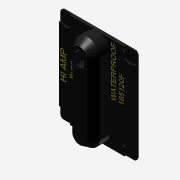
# Autodesk Inventor part: BUSS-COVER
Saved by Autodesk Inventor 2016 (Build 200138000, 138)
## iProperties
Shininess: 64.0
Length Units: 11272
Angle Units: 11279
Time Units: 11290
Mass Units: 11286
Length Display Precision: 3
Angle Display Precision: 2
Compacted: True
Part Number: BUSS-COVER
Document SubType Name: Modeling
Created: 2003-01-10
Designer: geyerm
Density: 1 g/cm^3
Material: Generic
Appearance: Glossy - Black
Mass: 7.12419 g
Surface Area: 49.8471 cm^2
Volume: 7.12419 cm^3
Density: 0.0
Volumn: 0.0
Area: 0.0
PropertySet Name: Model Information
Control State: 0
Master: False
Checked Out: False
Author: Autodesk
Autodesk Inventor part; units mm, degrees
ref_plane "YZ Plane" through (0, 0, 0) normal (1, 0, 0) x (0, 1, 0)
sketch "Sketch1" plane through (0, 0, 0) normal (0, 0, 1) x (1, 0, 0)
  arc A0 (-48.1199, -19.5796) -> (-46.5959, -21.1036) centre (-46.5959, -19.5796) ccw projected
  line L0 (-46.5959, -21.1036) -> (-10.7819, -21.1036) projected
  arc A1 (-10.7819, -21.1036) -> (-9.2579, -19.5796) centre (-10.7819, -19.5796) ccw projected
  line L1 (-9.2579, -19.5796) -> (-9.2579, 25.6324) projected
  arc A2 (-9.2579, 25.6324) -> (-10.7819, 27.1564) centre (-10.7819, 25.6324) ccw projected
  line L2 (-10.7819, 27.1564) -> (-46.5959, 27.1564) projected
  arc A3 (-46.5959, 27.1564) -> (-48.1199, 25.6324) centre (-46.5959, 25.6324) ccw projected
  line L3 (-48.1199, -19.5796) -> (-48.1199, 25.6324) projected
extrude "Extrusion1" add sketch "Sketch1" along normal blind 1.524
sketch "Sketch2" plane through (0, 0, 1.524) normal (0, 0, 1) x (1, 0, 0)
  line L0 (-10.7819, -21.1036) -> (-46.5959, -21.1036) projected
  line L1 (-46.5959, 27.1564) -> (-10.7819, 27.1564) projected
  line L2 (-35.0389, 20.8064) -> (-35.0389, -14.7536)
  arc A0 (-35.0389, -14.7536) -> (-22.3389, -14.7536) centre (-28.6889, -14.7536) ccw
  line L3 (-22.3389, -14.7536) -> (-22.3389, 20.8064)
  arc A1 (-22.3389, 20.8064) -> (-35.0389, 20.8064) centre (-28.6889, 20.8064) ccw
  line L4 (-28.6889, 27.1564) -> (-28.6889, -21.1036) construction
  dimension "d2" = 6.35
  constraints: 6 end point, 6 tangent, 4 point on circle, 2 centre point, 2 midpoint, 1 parallel, 1 point on line, 1 vertical
  measures "d2" radius of A1
extrude "Extrusion2" add sketch "Sketch2" along normal blind 8.89
chamfer "Chamfer2" distance 3.81 distance2 2.54 4 edges at (-35.0389, 3.0264, 10.414) (-28.6889, 27.1564, 10.414) (-22.3389, 3.0264, 10.414) (-28.6889, -21.1036, 10.414) measured on face at (-30.8056, 8.9531, 10.414) measured on face at (-35.0389, 8.9531, 4.4873)
sketch "Sketch3" plane through (0, 0, 10.414) normal (0, 0, 1) x (1, 0, 0)
  line L0 (-24.8789, 20.8064) -> (-24.8789, -14.7536) projected
  arc A0 (-24.8789, 20.8064) -> (-32.4989, 20.8064) centre (-28.6889, 20.8064) ccw projected
  line L1 (-30.8479, 20.8064) -> (-30.8479, 17.5044)
  arc A1 (-30.8479, 17.5044) -> (-26.5299, 17.5044) centre (-28.6889, 17.5044) ccw
  line L2 (-26.5299, 17.5044) -> (-26.5299, 20.8064)
  arc A2 (-26.5299, 20.8064) -> (-30.8479, 20.8064) centre (-28.6889, 20.8064) ccw
  dimension "d10" = 2.159
  dimension "d11" = 7.62
  constraints: 4 end point, 4 point on circle, 3 tangent, 2 centre point, 2 parallel, 1 coincident
  measures "d10" radius of A2
extrude "Extrusion3" cut sketch "Sketch3" against normal blind 8.89
ref_plane "Work Plane1" through (-48.1199, 3.0264, 0) normal (0, 1, 0) x (-1, 0, 0)
ref_plane "Work Plane2" through (-28.6889, 27.1564, 0) normal (1, 0, 0) x (0, 1, 0)
sketch "Sketch5" plane through (0, 0, 1.524) normal (0, 0, 1) x (1, 0, 0)
  line L0 (-35.0389, -14.7536) -> (-35.0389, 20.8064) projected
  line L1 (-46.5959, 27.1564) -> (-28.6889, 27.1564) projected
  arc A0 (-46.5959, 27.1564) -> (-48.1199, 25.6324) centre (-46.5959, 25.6324) ccw projected
  line L2 (-48.1199, -19.5796) -> (-48.1199, 25.6324) projected
  arc A1 (-47.0084, 21.5684) -> (-42.5319, 26.0449) centre (-44.9449, 23.9814) ccw
  line L3 (-41.7699, 23.9814) -> (-41.7699, 27.1564) construction
  line L4 (-44.9449, 20.8064) -> (-48.1199, 20.8064) construction
  line L5 (-47.0084, 21.5684) -> (-48.1199, 21.5684)
  line L6 (-42.5319, 26.0449) -> (-42.5319, 27.1564)
  dimension "d17" = 6.35
  dimension "d18" = 0.762
  dimension "d19" = 0.762
  constraints: 8 end point, 4 point on circle, 4 point on line, 4 tangent, 3 parallel, 1 centre point, 1 perpendicular
  measures "d17" diameter of A1
  measures "d18" distance between parallel lines of L6 L3
  measures "d19" distance between parallel lines of L5 L4
extrude "Extrusion5" cut sketch "Sketch5" against normal blind 0.762
mirror "Mirror3" about plane through (-48.1199, 3.0264, 0) normal (0, 1, 0) of "Extrusion5"
mirror "Mirror4" about plane through (-28.6889, 27.1564, 0) normal (1, 0, 0) of "Extrusion5", "Mirror3"
sketch "Sketch6" plane through (0, 0, 1.524) normal (0, 0, 1) x (1, 0, 0)
  line L0 (-48.1199, -15.5156) -> (-48.1199, 21.5684) projected
  line L1 (-47.3926, -5.3988) -> (-47.3926, 12.5954) construction
  line L2 (-47.3926, 12.5954) -> (-36.8812, 12.5954) construction
  line L3 (-36.8812, 12.5954) -> (-36.8812, -5.3988) construction
  line L4 (-36.8812, -5.3988) -> (-47.3926, -5.3988) construction
  line L5 (-44.3446, -3.3933) -> (-47.3926, -3.3933)
  line L6 (-47.3926, -3.3933) -> (-47.3926, -2.9891)
  line L7 (-47.3926, -2.9891) -> (-46.1404, -2.9891)
  line L8 (-46.1404, -2.9891) -> (-46.1404, -1.4093)
  line L9 (-46.1404, -1.4093) -> (-47.3926, -1.4093)
  line L10 (-47.3926, -1.4093) -> (-47.3926, -1.0051)
  line L11 (-47.3926, -1.0051) -> (-44.3446, -1.0051)
  line L12 (-44.3446, -1.0051) -> (-44.3446, -1.4093)
  line L13 (-44.3446, -1.4093) -> (-45.7803, -1.4093)
  line L14 (-45.7803, -1.4093) -> (-45.7803, -2.9891)
  line L15 (-45.7803, -2.9891) -> (-44.3446, -2.9891)
  line L16 (-44.3446, -2.9891) -> (-44.3446, -3.3933)
  line L17 (-44.3446, -0.264) -> (-47.3926, -0.264)
  line L18 (-47.3926, -0.264) -> (-47.3926, 0.1403)
  line L19 (-47.3926, 0.1403) -> (-44.3446, 0.1403)
  line L20 (-44.3446, 0.1403) -> (-44.3446, -0.264)
  line L21 (-44.3446, 1.6991) -> (-47.3926, 2.87)
  line L22 (-47.3926, 2.87) -> (-47.3926, 3.3067)
  line L23 (-47.3926, 3.3067) -> (-44.3446, 4.552)
  line L24 (-44.3446, 4.552) -> (-44.3446, 4.092)
  line L25 (-44.3446, 4.092) -> (-45.2669, 3.7388)
  line L26 (-45.2669, 3.7388) -> (-45.2669, 2.4611)
  line L27 (-45.2669, 2.4611) -> (-44.3446, 2.1266)
  line L28 (-44.3446, 2.1266) -> (-44.3446, 1.6991)
  line L29 (-45.5945, 2.5773) -> (-45.5945, 3.6134)
  line L30 (-45.5945, 3.6134) -> (-46.4401, 3.2928)
  spline S0 degree 2 poles (-46.4401, 3.2928) (-46.8257, 3.1488) (-47.072, 3.0791) knots 0 0 0 1 1 1
  spline S1 degree 2 poles (-47.072, 3.0791) (-46.7793, 3.0187) (-46.4889, 2.9141) knots 0 0 0 1 1 1
  line L31 (-46.4889, 2.9141) -> (-45.5945, 2.5773)
  line L32 (-44.3446, 4.8609) -> (-47.3926, 4.8609)
  line L33 (-47.3926, 4.8609) -> (-47.3926, 5.4673)
  line L34 (-47.3926, 5.4673) -> (-45.2344, 6.1898)
  spline S2 degree 2 poles (-45.2344, 6.1898) (-44.9324, 6.2897) (-44.7837, 6.3361) knots 0 0 0 1 1 1
  spline S3 degree 2 poles (-44.7837, 6.3361) (-44.9486, 6.3873) (-45.2715, 6.4988) knots 0 0 0 1 1 1
  line L35 (-45.2715, 6.4988) -> (-47.3926, 7.2306)
  line L36 (-47.3926, 7.2306) -> (-47.3926, 7.7719)
  line L37 (-47.3926, 7.7719) -> (-44.3446, 7.7719)
  line L38 (-44.3446, 7.7719) -> (-44.3446, 7.3839)
  line L39 (-44.3446, 7.3839) -> (-46.8954, 7.3839)
  line L40 (-46.8954, 7.3839) -> (-44.3446, 6.4941)
  line L41 (-44.3446, 6.4941) -> (-44.3446, 6.1317)
  line L42 (-44.3446, 6.1317) -> (-46.9396, 5.2489)
  line L43 (-46.9396, 5.2489) -> (-44.3446, 5.2489)
  line L44 (-44.3446, 5.2489) -> (-44.3446, 4.8609)
  line L45 (-44.3446, 8.42) -> (-47.3926, 8.42)
  line L46 (-47.3926, 8.42) -> (-47.3926, 9.57)
  spline S4 degree 2 poles (-47.3926, 9.57) (-47.3926, 9.8743) (-47.3624, 10.0346) knots 0 0 0 1 1 1
  spline S5 degree 4 poles (-47.3624, 10.0346) (-47.3252, 10.26) (-47.1161, 10.562) (-46.7375, 10.7478) (-46.5098, 10.7478) knots 0 0 0 0 0 1 1 1 1 1
  spline S6 degree 3 poles (-46.5098, 10.7478) (-46.1218, 10.7478) (-45.5829, 10.253) (-45.5829, 9.6072) knots 0 0 0 0 1 1 1 1
  line L47 (-45.5829, 9.6072) -> (-45.5829, 8.8243)
  line L48 (-45.5829, 8.8243) -> (-44.3446, 8.8243)
  line L49 (-44.3446, 8.8243) -> (-44.3446, 8.42)
  line L50 (-45.9429, 8.8243) -> (-45.9429, 9.6118)
  spline S7 degree 3 poles (-45.9429, 9.6118) (-45.9429, 10.0044) (-46.2333, 10.332) (-46.4982, 10.332) knots 0 0 0 0 1 1 1 1
  spline S8 degree 3 poles (-46.4982, 10.332) (-46.6887, 10.332) (-46.9628, 10.1392) (-47.0046, 9.9812) knots 0 0 0 0 1 1 1 1
  spline S9 degree 2 poles (-47.0046, 9.9812) (-47.0325, 9.879) (-47.0325, 9.6048) knots 0 0 0 1 1 1
  line L51 (-47.0325, 9.6048) -> (-47.0325, 8.8243)
  line L52 (-47.0325, 8.8243) -> (-45.9429, 8.8243)
  line L53 (-40.1526, -0.0878) -> (-42.6926, -0.0878)
  line L54 (-42.6926, -0.0878) -> (-42.6926, 0.8647)
  spline S10 degree 4 poles (-42.6926, 0.8647) (-42.6926, 1.1551) (-42.5378, 1.5074) (-42.2183, 1.7068) (-42.0421, 1.7068) knots 0 0 0 0 0 1 1 1 1 1
  spline S11 degree 3 poles (-42.0421, 1.7068) (-41.8795, 1.7068) (-41.593, 1.5307) (-41.5039, 1.3506) knots 0 0 0 0 1 1 1 1
  spline S12 degree 3 poles (-41.5039, 1.3506) (-41.4362, 1.5829) (-41.1109, 1.8307) (-40.8883, 1.8307) knots 0 0 0 0 1 1 1 1
  spline S13 degree 5 poles (-40.8883, 1.8307) (-40.7102, 1.8307) (-40.4043, 1.6797) (-40.2378, 1.459) (-40.1526, 1.1241) (-40.1526, 0.8802) knots 0 0 0 0 0 0 1 1 1 1 1 1
  line L55 (-40.1526, 0.8802) -> (-40.1526, -0.0878)
  line L56 (-40.4527, 0.2491) -> (-40.4527, 0.8821)
  spline S14 degree 2 poles (-40.4527, 0.8821) (-40.4527, 1.0447) (-40.4643, 1.1106) knots 0 0 0 1 1 1
  spline S15 degree 4 poles (-40.4643, 1.1106) (-40.4856, 1.2267) (-40.5824, 1.3835) (-40.7683, 1.4842) (-40.8902, 1.4842) knots 0 0 0 0 0 1 1 1 1 1
  spline S16 degree 4 poles (-40.8902, 1.4842) (-41.0316, 1.4842) (-41.2407, 1.3351) (-41.3258, 1.0776) (-41.3258, 0.8357) knots 0 0 0 0 0 1 1 1 1 1
  line L57 (-41.3258, 0.8357) -> (-41.3258, 0.2491)
  line L58 (-41.3258, 0.2491) -> (-40.4527, 0.2491)
  line L59 (-41.6259, 0.2491) -> (-41.6259, 0.7969)
  spline S17 degree 2 poles (-41.6259, 0.7969) (-41.6259, 1.0215) (-41.655, 1.1183) knots 0 0 0 1 1 1
  spline S18 degree 3 poles (-41.655, 1.1183) (-41.6937, 1.2461) (-41.8698, 1.3758) (-42.0034, 1.3758) knots 0 0 0 0 1 1 1 1
  spline S19 degree 4 poles (-42.0034, 1.3758) (-42.1293, 1.3758) (-42.3209, 1.2538) (-42.3926, 1.0293) (-42.3926, 0.7563) knots 0 0 0 0 0 1 1 1 1 1
  line L60 (-42.3926, 0.7563) -> (-42.3926, 0.2491)
  line L61 (-42.3926, 0.2491) -> (-41.6259, 0.2491)
  line L62 (-40.1526, 3.4589) -> (-40.4237, 3.4589)
  spline S20 degree 2 poles (-40.4237, 3.4589) (-40.112, 3.244) (-40.112, 2.8762) knots 0 0 0 1 1 1
  spline S21 degree 4 poles (-40.112, 2.8762) (-40.112, 2.7135) (-40.2359, 2.4309) (-40.4256, 2.2934) (-40.5631, 2.2663) knots 0 0 0 0 0 1 1 1 1 1
  spline S22 degree 2 poles (-40.5631, 2.2663) (-40.6541, 2.247) (-40.8535, 2.247) knots 0 0 0 1 1 1
  line L63 (-40.8535, 2.247) -> (-41.9937, 2.247)
  line L64 (-41.9937, 2.247) -> (-41.9937, 2.5587)
  line L65 (-41.9937, 2.5587) -> (-40.9735, 2.5587)
  spline S23 degree 2 poles (-40.9735, 2.5587) (-40.7296, 2.5587) (-40.6444, 2.578) knots 0 0 0 1 1 1
  spline S24 degree 3 poles (-40.6444, 2.578) (-40.5205, 2.6071) (-40.3811, 2.7968) (-40.3811, 2.9381) knots 0 0 0 0 1 1 1 1
  spline S25 degree 4 poles (-40.3811, 2.9381) (-40.3811, 3.0775) (-40.5243, 3.3234) (-40.7721, 3.426) (-41.0083, 3.426) knots 0 0 0 0 0 1 1 1 1 1
  line L66 (-41.0083, 3.426) -> (-41.9937, 3.426)
  line L67 (-41.9937, 3.426) -> (-41.9937, 3.7377)
  line L68 (-41.9937, 3.7377) -> (-40.1526, 3.7377)
  line L69 (-40.1526, 3.7377) -> (-40.1526, 3.4589)
  line L70 (-40.7025, 4.1016) -> (-40.7509, 4.4095)
  spline S26 degree 3 poles (-40.7509, 4.4095) (-40.565, 4.4346) (-40.3675, 4.6728) (-40.3675, 4.8876) knots 0 0 0 0 1 1 1 1
  spline S27 degree 3 poles (-40.3675, 4.8876) (-40.3675, 5.1025) (-40.5437, 5.3116) (-40.6618, 5.3116) knots 0 0 0 0 1 1 1 1
  spline S28 degree 2 poles (-40.6618, 5.3116) (-40.7663, 5.3116) (-40.8283, 5.2187) knots 0 0 0 1 1 1
  spline S29 degree 2 poles (-40.8283, 5.2187) (-40.8689, 5.1548) (-40.9328, 4.8993) knots 0 0 0 1 1 1
  spline S30 degree 4 poles (-40.9328, 4.8993) (-41.02, 4.5566) (-41.1458, 4.2914) (-41.3704, 4.1539) (-41.5039, 4.1539) knots 0 0 0 0 0 1 1 1 1 1
  spline S31 degree 3 poles (-41.5039, 4.1539) (-41.6278, 4.1539) (-41.8369, 4.2662) (-41.9066, 4.363) knots 0 0 0 0 1 1 1 1
  spline S32 degree 3 poles (-41.9066, 4.363) (-41.9608, 4.4366) (-42.0344, 4.6882) (-42.0344, 4.8334) knots 0 0 0 0 1 1 1 1
  spline S33 degree 4 poles (-42.0344, 4.8334) (-42.0344, 5.0503) (-41.9086, 5.3775) (-41.6956, 5.5343) (-41.5175, 5.5633) knots 0 0 0 0 0 1 1 1 1 1
  line L71 (-41.5175, 5.5633) -> (-41.4768, 5.2574)
  spline S34 degree 3 poles (-41.4768, 5.2574) (-41.6201, 5.2361) (-41.7789, 5.0367) (-41.7789, 4.8547) knots 0 0 0 0 1 1 1 1
  spline S35 degree 3 poles (-41.7789, 4.8547) (-41.7789, 4.6398) (-41.6356, 4.4559) (-41.5407, 4.4559) knots 0 0 0 0 1 1 1 1
  spline S36 degree 2 poles (-41.5407, 4.4559) (-41.4807, 4.4559) (-41.4323, 4.4946) knots 0 0 0 1 1 1
  spline S37 degree 2 poles (-41.4323, 4.4946) (-41.382, 4.5314) (-41.3491, 4.6147) knots 0 0 0 1 1 1
  spline S38 degree 2 poles (-41.3491, 4.6147) (-41.3316, 4.6611) (-41.2678, 4.8896) knots 0 0 0 1 1 1
  spline S39 degree 4 poles (-41.2678, 4.8896) (-41.1806, 5.2206) (-41.0684, 5.4839) (-40.8535, 5.633) (-40.6928, 5.633) knots 0 0 0 0 0 1 1 1 1 1
  spline S40 degree 4 poles (-40.6928, 5.633) (-40.5379, 5.633) (-40.263, 5.451) (-40.112, 5.1064) (-40.112, 4.8896) knots 0 0 0 0 0 1 1 1 1 1
  spline S41 degree 3 poles (-40.112, 4.8896) (-40.112, 4.5314) (-40.4101, 4.1539) (-40.7025, 4.1016) knots 0 0 0 0 1 1 1 1
  line L72 (-40.7025, 5.8769) -> (-40.7509, 6.1848)
  spline S42 degree 3 poles (-40.7509, 6.1848) (-40.565, 6.2099) (-40.3675, 6.448) (-40.3675, 6.6629) knots 0 0 0 0 1 1 1 1
  spline S43 degree 3 poles (-40.3675, 6.6629) (-40.3675, 6.8778) (-40.5437, 7.0869) (-40.6618, 7.0869) knots 0 0 0 0 1 1 1 1
  spline S44 degree 2 poles (-40.6618, 7.0869) (-40.7663, 7.0869) (-40.8283, 6.994) knots 0 0 0 1 1 1
  spline S45 degree 2 poles (-40.8283, 6.994) (-40.8689, 6.9301) (-40.9328, 6.6746) knots 0 0 0 1 1 1
  spline S46 degree 4 poles (-40.9328, 6.6746) (-41.02, 6.3319) (-41.1458, 6.0667) (-41.3704, 5.9292) (-41.5039, 5.9292) knots 0 0 0 0 0 1 1 1 1 1
  spline S47 degree 3 poles (-41.5039, 5.9292) (-41.6278, 5.9292) (-41.8369, 6.0415) (-41.9066, 6.1383) knots 0 0 0 0 1 1 1 1
  spline S48 degree 3 poles (-41.9066, 6.1383) (-41.9608, 6.2119) (-42.0344, 6.4635) (-42.0344, 6.6087) knots 0 0 0 0 1 1 1 1
  spline S49 degree 4 poles (-42.0344, 6.6087) (-42.0344, 6.8256) (-41.9086, 7.1527) (-41.6956, 7.3096) (-41.5175, 7.3386) knots 0 0 0 0 0 1 1 1 1 1
  line L73 (-41.5175, 7.3386) -> (-41.4768, 7.0327)
  spline S50 degree 3 poles (-41.4768, 7.0327) (-41.6201, 7.0114) (-41.7789, 6.812) (-41.7789, 6.63) knots 0 0 0 0 1 1 1 1
  spline S51 degree 3 poles (-41.7789, 6.63) (-41.7789, 6.4151) (-41.6356, 6.2312) (-41.5407, 6.2312) knots 0 0 0 0 1 1 1 1
  spline S52 degree 2 poles (-41.5407, 6.2312) (-41.4807, 6.2312) (-41.4323, 6.2699) knots 0 0 0 1 1 1
  spline S53 degree 2 poles (-41.4323, 6.2699) (-41.382, 6.3067) (-41.3491, 6.39) knots 0 0 0 1 1 1
  spline S54 degree 2 poles (-41.3491, 6.39) (-41.3316, 6.4364) (-41.2678, 6.6649) knots 0 0 0 1 1 1
  spline S55 degree 4 poles (-41.2678, 6.6649) (-41.1806, 6.9959) (-41.0684, 7.2592) (-40.8535, 7.4083) (-40.6928, 7.4083) knots 0 0 0 0 0 1 1 1 1 1
  spline S56 degree 4 poles (-40.6928, 7.4083) (-40.5379, 7.4083) (-40.263, 7.2263) (-40.112, 6.8817) (-40.112, 6.6649) knots 0 0 0 0 0 1 1 1 1 1
  spline S57 degree 3 poles (-40.112, 6.6649) (-40.112, 6.3067) (-40.4101, 5.9292) (-40.7025, 5.8769) knots 0 0 0 0 1 1 1 1
  line L74 (-36.1554, 0.7708) -> (-36.1554, 0.4591)
  line L75 (-36.1554, 0.4591) -> (-38.1417, 0.4591)
  spline S58 degree 3 poles (-38.1417, 0.4591) (-38.0353, 0.3468) (-37.8204, -0.0191) (-37.7662, -0.1643) knots 0 0 0 0 1 1 1 1
  line L76 (-37.7662, -0.1643) -> (-38.0682, -0.1643)
  spline S59 degree 3 poles (-38.0682, -0.1643) (-38.1901, 0.0971) (-38.5406, 0.4881) (-38.7051, 0.5695) knots 0 0 0 0 1 1 1 1
  line L77 (-38.7051, 0.5695) -> (-38.7051, 0.7708)
  line L78 (-38.7051, 0.7708) -> (-36.1554, 0.7708)
  line L79 (-36.4555, 3.2082) -> (-36.1554, 3.2082)
  line L80 (-36.1554, 3.2082) -> (-36.1554, 1.5297)
  spline S60 degree 2 poles (-36.1554, 1.5297) (-36.2677, 1.5258) (-36.3723, 1.5665) knots 0 0 0 1 1 1
  spline S61 degree 3 poles (-36.3723, 1.5665) (-36.5446, 1.6304) (-36.8756, 1.913) (-37.0944, 2.1802) knots 0 0 0 0 1 1 1 1
  spline S62 degree 3 poles (-37.0944, 2.1802) (-37.4351, 2.5926) (-37.83, 2.8829) (-38.0082, 2.8829) knots 0 0 0 0 1 1 1 1
  spline S63 degree 3 poles (-38.0082, 2.8829) (-38.194, 2.8829) (-38.4476, 2.6177) (-38.4476, 2.4048) knots 0 0 0 0 1 1 1 1
  spline S64 degree 3 poles (-38.4476, 2.4048) (-38.4476, 2.1802) (-38.1766, 1.9111) (-37.9385, 1.9092) knots 0 0 0 0 1 1 1 1
  line L81 (-37.9385, 1.9092) -> (-37.9714, 1.5878)
  spline S65 degree 3 poles (-37.9714, 1.5878) (-38.3295, 1.6207) (-38.7051, 2.0505) (-38.7051, 2.4125) knots 0 0 0 0 1 1 1 1
  spline S66 degree 3 poles (-38.7051, 2.4125) (-38.7051, 2.7784) (-38.3005, 3.2043) (-38.0004, 3.2043) knots 0 0 0 0 1 1 1 1
  spline S67 degree 4 poles (-38.0004, 3.2043) (-37.8475, 3.2043) (-37.5532, 3.0804) (-37.228, 2.79) (-36.9434, 2.4551) knots 0 0 0 0 0 1 1 1 1 1
  spline S68 degree 3 poles (-36.9434, 2.4551) (-36.7091, 2.1744) (-36.5407, 2.0156) (-36.4555, 1.9634) knots 0 0 0 0 1 1 1 1
  line L82 (-36.4555, 1.9634) -> (-36.4555, 3.2082)
  spline S69 degree 4 poles (-37.408, 3.5431) (-37.8591, 3.5431) (-38.4089, 3.729) (-38.7051, 4.0929) (-38.7051, 4.3717) knots 0 0 0 0 0 1 1 1 1 1
  spline S70 degree 5 poles (-38.7051, 4.3717) (-38.7051, 4.575) (-38.5406, 4.8847) (-38.2308, 5.0842) (-37.7855, 5.1984) (-37.408, 5.1984) knots 0 0 0 0 0 0 1 1 1 1 1 1
  spline S71 degree 4 poles (-37.408, 5.1984) (-36.9608, 5.1984) (-36.411, 5.0145) (-36.1128, 4.6486) (-36.1128, 4.3717) knots 0 0 0 0 0 1 1 1 1 1
  spline S72 degree 2 poles (-36.1128, 4.3717) (-36.1128, 4.0039) (-36.3742, 3.7948) knots 0 0 0 1 1 1
  spline S73 degree 2 poles (-36.3742, 3.7948) (-36.6936, 3.5431) (-37.408, 3.5431) knots 0 0 0 1 1 1
  spline S74 degree 3 poles (-37.408, 3.8645) (-36.7808, 3.8645) (-36.3684, 4.1568) (-36.3684, 4.3717) knots 0 0 0 0 1 1 1 1
  spline S75 degree 3 poles (-36.3684, 4.3717) (-36.3684, 4.5847) (-36.7827, 4.877) (-37.408, 4.877) knots 0 0 0 0 1 1 1 1
  spline S76 degree 3 poles (-37.408, 4.877) (-38.0353, 4.877) (-38.4476, 4.5847) (-38.4476, 4.3678) knots 0 0 0 0 1 1 1 1
  spline S77 degree 2 poles (-38.4476, 4.3678) (-38.4476, 4.1529) (-38.2656, 4.0252) knots 0 0 0 1 1 1
  spline S78 degree 2 poles (-38.2656, 4.0252) (-38.0333, 3.8645) (-37.408, 3.8645) knots 0 0 0 1 1 1
  line L83 (-36.1554, 5.3649) -> (-38.6954, 6.3406)
  line L84 (-38.6954, 6.3406) -> (-38.6954, 6.7046)
  line L85 (-38.6954, 6.7046) -> (-36.1554, 7.7422)
  line L86 (-36.1554, 7.7422) -> (-36.1554, 7.3589)
  line L87 (-36.1554, 7.3589) -> (-36.924, 7.0647)
  line L88 (-36.924, 7.0647) -> (-36.924, 5.9999)
  line L89 (-36.924, 5.9999) -> (-36.1554, 5.7211)
  line L90 (-36.1554, 5.7211) -> (-36.1554, 5.3649)
  line L91 (-37.197, 6.0967) -> (-37.197, 6.9601)
  line L92 (-37.197, 6.9601) -> (-37.9017, 6.6929)
  spline S79 degree 2 poles (-37.9017, 6.6929) (-38.2231, 6.5729) (-38.4283, 6.5148) knots 0 0 0 1 1 1
  spline S80 degree 2 poles (-38.4283, 6.5148) (-38.1843, 6.4645) (-37.9423, 6.3774) knots 0 0 0 1 1 1
  line L93 (-37.9423, 6.3774) -> (-37.197, 6.0967)
  constraints: 1 parallel, 2 other
emboss "Emboss1" sketch "Sketch6" operation add depth 0.0508 direction (0, 0, -1)
sketch "Sketch7" plane through (0, 0, 1.524) normal (0, 0, 1) x (1, 0, 0)
  line L0 (-9.2579, 21.5684) -> (-9.2579, -15.5156) projected
  line L1 (-21.7032, 0.6221) -> (-21.7032, 0.6221) construction
  line L2 (-21.7032, 0.6221) -> (-21.7032, 0.6221) construction
  line L3 (-21.7032, 0.6221) -> (-21.7032, 0.6221) construction
  line L4 (-21.7032, 0.6221) -> (-21.7032, 0.6221) construction
  line L5 (-19.1186, 1.3384) -> (-21.6586, 0.6647)
  line L6 (-21.6586, 0.6647) -> (-21.6586, 1.0093)
  line L7 (-21.6586, 1.0093) -> (-19.9937, 1.3965)
  spline S0 degree 2 poles (-19.9937, 1.3965) (-19.7323, 1.4584) (-19.4729, 1.5049) knots 0 0 0 1 1 1
  spline S1 degree 2 poles (-19.4729, 1.5049) (-19.8814, 1.6017) (-19.9434, 1.6191) knots 0 0 0 1 1 1
  line L8 (-19.9434, 1.6191) -> (-21.6586, 2.1012)
  line L9 (-21.6586, 2.1012) -> (-21.6586, 2.5077)
  line L10 (-21.6586, 2.5077) -> (-20.3732, 2.8717)
  spline S2 degree 2 poles (-20.3732, 2.8717) (-19.895, 3.0053) (-19.4729, 3.0692) knots 0 0 0 1 1 1
  spline S3 degree 2 poles (-19.4729, 3.0692) (-19.7149, 3.1176) (-20.0266, 3.195) knots 0 0 0 1 1 1
  line L11 (-20.0266, 3.195) -> (-21.6586, 3.5919)
  line L12 (-21.6586, 3.5919) -> (-21.6586, 3.9307)
  line L13 (-21.6586, 3.9307) -> (-19.1186, 3.2376)
  line L14 (-19.1186, 3.2376) -> (-19.1186, 2.9085)
  line L15 (-19.1186, 2.9085) -> (-21.0546, 2.378)
  spline S4 degree 2 poles (-21.0546, 2.378) (-21.2966, 2.3083) (-21.3528, 2.2967) knots 0 0 0 1 1 1
  spline S5 degree 2 poles (-21.3528, 2.2967) (-21.1785, 2.2541) (-21.0546, 2.2212) knots 0 0 0 1 1 1
  line L16 (-21.0546, 2.2212) -> (-19.1186, 1.6849)
  line L17 (-19.1186, 1.6849) -> (-19.1186, 1.3384)
  line L18 (-19.1186, 3.9674) -> (-21.6586, 4.9432)
  line L19 (-21.6586, 4.9432) -> (-21.6586, 5.3071)
  line L20 (-21.6586, 5.3071) -> (-19.1186, 6.3448)
  line L21 (-19.1186, 6.3448) -> (-19.1186, 5.9615)
  line L22 (-19.1186, 5.9615) -> (-19.8872, 5.6672)
  line L23 (-19.8872, 5.6672) -> (-19.8872, 4.6024)
  line L24 (-19.8872, 4.6024) -> (-19.1186, 4.3237)
  line L25 (-19.1186, 4.3237) -> (-19.1186, 3.9674)
  line L26 (-20.1602, 4.6992) -> (-20.1602, 5.5627)
  line L27 (-20.1602, 5.5627) -> (-20.8649, 5.2955)
  spline S6 degree 2 poles (-20.8649, 5.2955) (-21.1863, 5.1755) (-21.3915, 5.1174) knots 0 0 0 1 1 1
  spline S7 degree 2 poles (-21.3915, 5.1174) (-21.1475, 5.0671) (-20.9055, 4.98) knots 0 0 0 1 1 1
  line L28 (-20.9055, 4.98) -> (-20.1602, 4.6992)
  line L29 (-19.1186, 7.2586) -> (-21.3586, 7.2586)
  line L30 (-21.3586, 7.2586) -> (-21.3586, 6.4223)
  line L31 (-21.3586, 6.4223) -> (-21.6586, 6.4223)
  line L32 (-21.6586, 6.4223) -> (-21.6586, 8.4357)
  line L33 (-21.6586, 8.4357) -> (-21.3586, 8.4357)
  line L34 (-21.3586, 8.4357) -> (-21.3586, 7.5955)
  line L35 (-21.3586, 7.5955) -> (-19.1186, 7.5955)
  line L36 (-19.1186, 7.5955) -> (-19.1186, 7.2586)
  line L37 (-19.1186, 8.788) -> (-21.6586, 8.788)
  line L38 (-21.6586, 8.788) -> (-21.6586, 10.6272)
  line L39 (-21.6586, 10.6272) -> (-21.3586, 10.6272)
  line L40 (-21.3586, 10.6272) -> (-21.3586, 9.1249)
  line L41 (-21.3586, 9.1249) -> (-20.5822, 9.1249)
  line L42 (-20.5822, 9.1249) -> (-20.5822, 10.5323)
  line L43 (-20.5822, 10.5323) -> (-20.2822, 10.5323)
  line L44 (-20.2822, 10.5323) -> (-20.2822, 9.1249)
  line L45 (-20.2822, 9.1249) -> (-19.4187, 9.1249)
  line L46 (-19.4187, 9.1249) -> (-19.4187, 10.6853)
  line L47 (-19.4187, 10.6853) -> (-19.1186, 10.6853)
  line L48 (-19.1186, 10.6853) -> (-19.1186, 8.788)
  line L49 (-19.1186, 11.1538) -> (-21.6586, 11.1538)
  line L50 (-21.6586, 11.1538) -> (-21.6586, 12.2805)
  spline S8 degree 4 poles (-21.6586, 12.2805) (-21.6586, 12.6193) (-21.5212, 12.9736) (-21.1746, 13.1846) (-20.9656, 13.1846) knots 0 0 0 0 0 1 1 1 1 1
  spline S9 degree 3 poles (-20.9656, 13.1846) (-20.6945, 13.1846) (-20.3248, 12.8342) (-20.2744, 12.4703) knots 0 0 0 0 1 1 1 1
  spline S10 degree 2 poles (-20.2744, 12.4703) (-20.2105, 12.6019) (-20.1486, 12.6716) knots 0 0 0 1 1 1
  spline S11 degree 2 poles (-20.1486, 12.6716) (-20.0131, 12.8187) (-19.8098, 12.9504) knots 0 0 0 1 1 1
  line L51 (-19.8098, 12.9504) -> (-19.1186, 13.3898)
  line L52 (-19.1186, 13.3898) -> (-19.1186, 12.9697)
  line L53 (-19.1186, 12.9697) -> (-19.6472, 12.6329)
  spline S12 degree 4 poles (-19.6472, 12.6329) (-19.8756, 12.4857) (-20.1176, 12.296) (-20.2163, 12.145) (-20.2357, 12.0676) knots 0 0 0 0 0 1 1 1 1 1
  spline S13 degree 2 poles (-20.2357, 12.0676) (-20.2473, 12.0095) (-20.2473, 11.8798) knots 0 0 0 1 1 1
  line L54 (-20.2473, 11.8798) -> (-20.2473, 11.4906)
  line L55 (-20.2473, 11.4906) -> (-19.1186, 11.4906)
  line L56 (-19.1186, 11.4906) -> (-19.1186, 11.1538)
  line L57 (-20.5377, 11.4906) -> (-20.5377, 12.2128)
  spline S14 degree 4 poles (-20.5377, 12.2128) (-20.5377, 12.4431) (-20.6326, 12.7026) (-20.8436, 12.8381) (-20.9656, 12.8381) knots 0 0 0 0 0 1 1 1 1 1
  spline S15 degree 3 poles (-20.9656, 12.8381) (-21.1456, 12.8381) (-21.3779, 12.5767) (-21.3779, 12.2941) knots 0 0 0 0 1 1 1 1
  line L58 (-21.3779, 12.2941) -> (-21.3779, 11.4906)
  line L59 (-21.3779, 11.4906) -> (-20.5377, 11.4906)
  line L60 (-19.1186, 13.7112) -> (-21.6586, 13.7112)
  line L61 (-21.6586, 13.7112) -> (-21.6586, 14.6695)
  spline S16 degree 2 poles (-21.6586, 14.6695) (-21.6586, 14.9231) (-21.6335, 15.0567) knots 0 0 0 1 1 1
  spline S17 degree 4 poles (-21.6335, 15.0567) (-21.6025, 15.2445) (-21.4283, 15.4962) (-21.1127, 15.6511) (-20.923, 15.6511) knots 0 0 0 0 0 1 1 1 1 1
  spline S18 degree 3 poles (-20.923, 15.6511) (-20.5997, 15.6511) (-20.1505, 15.2387) (-20.1505, 14.7005) knots 0 0 0 0 1 1 1 1
  line L62 (-20.1505, 14.7005) -> (-20.1505, 14.0481)
  line L63 (-20.1505, 14.0481) -> (-19.1186, 14.0481)
  line L64 (-19.1186, 14.0481) -> (-19.1186, 13.7112)
  line L65 (-20.4506, 14.0481) -> (-20.4506, 14.7044)
  spline S19 degree 3 poles (-20.4506, 14.7044) (-20.4506, 15.0315) (-20.6926, 15.3045) (-20.9133, 15.3045) knots 0 0 0 0 1 1 1 1
  spline S20 degree 3 poles (-20.9133, 15.3045) (-21.072, 15.3045) (-21.3005, 15.1438) (-21.3353, 15.0122) knots 0 0 0 0 1 1 1 1
  spline S21 degree 2 poles (-21.3353, 15.0122) (-21.3586, 14.927) (-21.3586, 14.6986) knots 0 0 0 1 1 1
  line L66 (-21.3586, 14.6986) -> (-21.3586, 14.0481)
  line L67 (-21.3586, 14.0481) -> (-20.4506, 14.0481)
  line L68 (-19.1186, 16.0847) -> (-21.6586, 16.0847)
  line L69 (-21.6586, 16.0847) -> (-21.6586, 17.2115)
  spline S22 degree 4 poles (-21.6586, 17.2115) (-21.6586, 17.5503) (-21.5212, 17.9045) (-21.1746, 18.1156) (-20.9656, 18.1156) knots 0 0 0 0 0 1 1 1 1 1
  spline S23 degree 3 poles (-20.9656, 18.1156) (-20.6945, 18.1156) (-20.3248, 17.7651) (-20.2744, 17.4012) knots 0 0 0 0 1 1 1 1
  spline S24 degree 2 poles (-20.2744, 17.4012) (-20.2105, 17.5328) (-20.1486, 17.6025) knots 0 0 0 1 1 1
  spline S25 degree 2 poles (-20.1486, 17.6025) (-20.0131, 17.7497) (-19.8098, 17.8813) knots 0 0 0 1 1 1
  line L70 (-19.8098, 17.8813) -> (-19.1186, 18.3208)
  line L71 (-19.1186, 18.3208) -> (-19.1186, 17.9007)
  line L72 (-19.1186, 17.9007) -> (-19.6472, 17.5638)
  spline S26 degree 4 poles (-19.6472, 17.5638) (-19.8756, 17.4167) (-20.1176, 17.2269) (-20.2163, 17.0759) (-20.2357, 16.9985) knots 0 0 0 0 0 1 1 1 1 1
  spline S27 degree 2 poles (-20.2357, 16.9985) (-20.2473, 16.9404) (-20.2473, 16.8107) knots 0 0 0 1 1 1
  line L73 (-20.2473, 16.8107) -> (-20.2473, 16.4216)
  line L74 (-20.2473, 16.4216) -> (-19.1186, 16.4216)
  line L75 (-19.1186, 16.4216) -> (-19.1186, 16.0847)
  line L76 (-20.5377, 16.4216) -> (-20.5377, 17.1437)
  spline S28 degree 4 poles (-20.5377, 17.1437) (-20.5377, 17.3741) (-20.6326, 17.6335) (-20.8436, 17.769) (-20.9656, 17.769) knots 0 0 0 0 0 1 1 1 1 1
  spline S29 degree 3 poles (-20.9656, 17.769) (-21.1456, 17.769) (-21.3779, 17.5077) (-21.3779, 17.225) knots 0 0 0 0 1 1 1 1
  line L77 (-21.3779, 17.225) -> (-21.3779, 16.4216)
  line L78 (-21.3779, 16.4216) -> (-20.5377, 16.4216)
  spline S30 degree 3 poles (-20.3557, 18.5415) (-20.9888, 18.5415) (-21.7032, 19.221) (-21.7032, 19.7573) knots 0 0 0 0 1 1 1 1
  spline S31 degree 4 poles (-21.7032, 19.7573) (-21.7032, 20.1096) (-21.3663, 20.6749) (-20.7662, 20.9711) (-20.3848, 20.9711) knots 0 0 0 0 0 1 1 1 1 1
  spline S32 degree 4 poles (-20.3848, 20.9711) (-19.9995, 20.9711) (-19.3897, 20.6594) (-19.076, 20.0864) (-19.076, 19.7573) knots 0 0 0 0 0 1 1 1 1 1
  spline S33 degree 4 poles (-19.076, 19.7573) (-19.076, 19.3972) (-19.4226, 18.8319) (-20.0208, 18.5415) (-20.3557, 18.5415) knots 0 0 0 0 0 1 1 1 1 1
  spline S34 degree 3 poles (-20.3519, 18.888) (-19.893, 18.888) (-19.3645, 19.3817) (-19.3645, 19.7553) knots 0 0 0 0 1 1 1 1
  spline S35 degree 3 poles (-19.3645, 19.7553) (-19.3645, 20.1348) (-19.8969, 20.6246) (-20.3886, 20.6246) knots 0 0 0 0 1 1 1 1
  spline S36 degree 4 poles (-20.3886, 20.6246) (-20.6984, 20.6246) (-21.1611, 20.4155) (-21.4147, 20.0109) (-21.4147, 19.7592) knots 0 0 0 0 0 1 1 1 1 1
  spline S37 degree 3 poles (-21.4147, 19.7592) (-21.4147, 19.403) (-20.9249, 18.888) (-20.3519, 18.888) knots 0 0 0 0 1 1 1 1
  spline S38 degree 3 poles (-20.3557, 21.3022) (-20.9888, 21.3022) (-21.7032, 21.9817) (-21.7032, 22.518) knots 0 0 0 0 1 1 1 1
  spline S39 degree 4 poles (-21.7032, 22.518) (-21.7032, 22.8703) (-21.3663, 23.4356) (-20.7662, 23.7318) (-20.3848, 23.7318) knots 0 0 0 0 0 1 1 1 1 1
  spline S40 degree 4 poles (-20.3848, 23.7318) (-19.9995, 23.7318) (-19.3897, 23.4201) (-19.076, 22.8471) (-19.076, 22.518) knots 0 0 0 0 0 1 1 1 1 1
  spline S41 degree 4 poles (-19.076, 22.518) (-19.076, 22.1579) (-19.4226, 21.5926) (-20.0208, 21.3022) (-20.3557, 21.3022) knots 0 0 0 0 0 1 1 1 1 1
  spline S42 degree 3 poles (-20.3519, 21.6487) (-19.893, 21.6487) (-19.3645, 22.1424) (-19.3645, 22.516) knots 0 0 0 0 1 1 1 1
  spline S43 degree 3 poles (-19.3645, 22.516) (-19.3645, 22.8955) (-19.8969, 23.3853) (-20.3886, 23.3853) knots 0 0 0 0 1 1 1 1
  spline S44 degree 4 poles (-20.3886, 23.3853) (-20.6984, 23.3853) (-21.1611, 23.1762) (-21.4147, 22.7716) (-21.4147, 22.5199) knots 0 0 0 0 0 1 1 1 1 1
  spline S45 degree 3 poles (-21.4147, 22.5199) (-21.4147, 22.1637) (-20.9249, 21.6487) (-20.3519, 21.6487) knots 0 0 0 0 1 1 1 1
  line L79 (-19.1186, 24.181) -> (-21.6586, 24.181)
  line L80 (-21.6586, 24.181) -> (-21.6586, 25.8962)
  line L81 (-21.6586, 25.8962) -> (-21.3586, 25.8962)
  line L82 (-21.3586, 25.8962) -> (-21.3586, 24.5178)
  line L83 (-21.3586, 24.5178) -> (-20.5726, 24.5178)
  line L84 (-20.5726, 24.5178) -> (-20.5726, 25.7104)
  line L85 (-20.5726, 25.7104) -> (-20.2725, 25.7104)
  line L86 (-20.2725, 25.7104) -> (-20.2725, 24.5178)
  line L87 (-20.2725, 24.5178) -> (-19.1186, 24.5178)
  line L88 (-19.1186, 24.5178) -> (-19.1186, 24.181)
  line L89 (-15.1214, 1.9424) -> (-15.1214, 1.6307)
  line L90 (-15.1214, 1.6307) -> (-17.1077, 1.6307)
  spline S46 degree 3 poles (-17.1077, 1.6307) (-17.0013, 1.5184) (-16.7864, 1.1525) (-16.7322, 1.0073) knots 0 0 0 0 1 1 1 1
  line L91 (-16.7322, 1.0073) -> (-17.0342, 1.0073)
  spline S47 degree 3 poles (-17.0342, 1.0073) (-17.1561, 1.2687) (-17.5066, 1.6598) (-17.6711, 1.7411) knots 0 0 0 0 1 1 1 1
  line L92 (-17.6711, 1.7411) -> (-17.6711, 1.9424)
  line L93 (-17.6711, 1.9424) -> (-15.1214, 1.9424)
  spline S48 degree 3 poles (-16.4999, 3.224) (-16.5715, 3.0285) (-16.8348, 2.8407) (-17.0168, 2.8407) knots 0 0 0 0 1 1 1 1
  spline S49 degree 3 poles (-17.0168, 2.8407) (-17.2936, 2.8407) (-17.6711, 3.2395) (-17.6711, 3.5686) knots 0 0 0 0 1 1 1 1
  spline S50 degree 3 poles (-17.6711, 3.5686) (-17.6711, 3.9016) (-17.2859, 4.3062) (-17.009, 4.3062) knots 0 0 0 0 1 1 1 1
  spline S51 degree 3 poles (-17.009, 4.3062) (-16.8328, 4.3062) (-16.5715, 4.1204) (-16.4999, 3.9307) knots 0 0 0 0 1 1 1 1
  spline S52 degree 3 poles (-16.4999, 3.9307) (-16.4243, 4.1669) (-16.0836, 4.4108) (-15.8474, 4.4108) knots 0 0 0 0 1 1 1 1
  spline S53 degree 3 poles (-15.8474, 4.4108) (-15.5222, 4.4108) (-15.0788, 3.95) (-15.0788, 3.5744) knots 0 0 0 0 1 1 1 1
  spline S54 degree 3 poles (-15.0788, 3.5744) (-15.0788, 3.1989) (-15.5241, 2.7381) (-15.8571, 2.7381) knots 0 0 0 0 1 1 1 1
  spline S55 degree 3 poles (-15.8571, 2.7381) (-16.1049, 2.7381) (-16.4398, 2.9898) (-16.4999, 3.224) knots 0 0 0 0 1 1 1 1
  spline S56 degree 4 poles (-15.8552, 3.0595) (-15.7216, 3.0595) (-15.4718, 3.1853) (-15.3344, 3.4331) (-15.3344, 3.5764) knots 0 0 0 0 0 1 1 1 1 1
  spline S57 degree 3 poles (-15.3344, 3.5764) (-15.3344, 3.801) (-15.6229, 4.0894) (-15.8436, 4.0894) knots 0 0 0 0 1 1 1 1
  spline S58 degree 3 poles (-15.8436, 4.0894) (-16.0701, 4.0894) (-16.3643, 3.7913) (-16.3643, 3.5667) knots 0 0 0 0 1 1 1 1
  spline S59 degree 3 poles (-16.3643, 3.5667) (-16.3643, 3.346) (-16.0739, 3.0595) (-15.8552, 3.0595) knots 0 0 0 0 1 1 1 1
  spline S60 degree 3 poles (-17.0284, 3.1621) (-16.8483, 3.1621) (-16.6199, 3.3925) (-16.6199, 3.5764) knots 0 0 0 0 1 1 1 1
  spline S61 degree 3 poles (-16.6199, 3.5764) (-16.6199, 3.7564) (-16.8464, 3.9849) (-17.0109, 3.9849) knots 0 0 0 0 1 1 1 1
  spline S62 degree 3 poles (-17.0109, 3.9849) (-17.1813, 3.9849) (-17.4156, 3.7506) (-17.4156, 3.5744) knots 0 0 0 0 1 1 1 1
  spline S63 degree 3 poles (-17.4156, 3.5744) (-17.4156, 3.3944) (-17.1871, 3.1621) (-17.0284, 3.1621) knots 0 0 0 0 1 1 1 1
  line L94 (-15.7874, 4.7147) -> (-15.8145, 5.0419)
  spline S64 degree 3 poles (-15.8145, 5.0419) (-15.5745, 5.0787) (-15.3344, 5.342) (-15.3344, 5.5298) knots 0 0 0 0 1 1 1 1
  spline S65 degree 3 poles (-15.3344, 5.5298) (-15.3344, 5.7582) (-15.6751, 6.068) (-15.9558, 6.068) knots 0 0 0 0 1 1 1 1
  spline S66 degree 3 poles (-15.9558, 6.068) (-16.223, 6.068) (-16.5328, 5.7698) (-16.5328, 5.5259) knots 0 0 0 0 1 1 1 1
  spline S67 degree 3 poles (-16.5328, 5.5259) (-16.5328, 5.3749) (-16.3953, 5.1329) (-16.285, 5.0632) knots 0 0 0 0 1 1 1 1
  line L95 (-16.285, 5.0632) -> (-16.3237, 4.7709)
  line L96 (-16.3237, 4.7709) -> (-17.6285, 5.0167)
  line L97 (-17.6285, 5.0167) -> (-17.6285, 6.279)
  line L98 (-17.6285, 6.279) -> (-17.3304, 6.279)
  line L99 (-17.3304, 6.279) -> (-17.3304, 5.2665)
  line L100 (-17.3304, 5.2665) -> (-16.6489, 5.129)
  spline S68 degree 2 poles (-16.6489, 5.129) (-16.8077, 5.3575) (-16.8077, 5.6092) knots 0 0 0 1 1 1
  spline S69 degree 3 poles (-16.8077, 5.6092) (-16.8077, 5.9421) (-16.3469, 6.399) (-15.9849, 6.399) knots 0 0 0 0 1 1 1 1
  spline S70 degree 2 poles (-15.9849, 6.399) (-15.6383, 6.399) (-15.3867, 6.1977) knots 0 0 0 1 1 1
  spline S71 degree 2 poles (-15.3867, 6.1977) (-15.0788, 5.9538) (-15.0788, 5.5317) knots 0 0 0 1 1 1
  spline S72 degree 3 poles (-15.0788, 5.5317) (-15.0788, 5.1852) (-15.466, 4.7457) (-15.7874, 4.7147) knots 0 0 0 0 1 1 1 1
  line L101 (-15.1214, 7.8607) -> (-15.1214, 7.549)
  line L102 (-15.1214, 7.549) -> (-17.1077, 7.549)
  spline S73 degree 3 poles (-17.1077, 7.549) (-17.0013, 7.4367) (-16.7864, 7.0708) (-16.7322, 6.9256) knots 0 0 0 0 1 1 1 1
  line L103 (-16.7322, 6.9256) -> (-17.0342, 6.9256)
  spline S74 degree 3 poles (-17.0342, 6.9256) (-17.1561, 7.187) (-17.5066, 7.578) (-17.6711, 7.6594) knots 0 0 0 0 1 1 1 1
  line L104 (-17.6711, 7.6594) -> (-17.6711, 7.8607)
  line L105 (-17.6711, 7.8607) -> (-15.1214, 7.8607)
  line L106 (-15.4215, 10.2981) -> (-15.1214, 10.2981)
  line L107 (-15.1214, 10.2981) -> (-15.1214, 8.6196)
  spline S75 degree 2 poles (-15.1214, 8.6196) (-15.2337, 8.6157) (-15.3383, 8.6564) knots 0 0 0 1 1 1
  spline S76 degree 3 poles (-15.3383, 8.6564) (-15.5106, 8.7203) (-15.8416, 9.0029) (-16.0604, 9.2701) knots 0 0 0 0 1 1 1 1
  spline S77 degree 3 poles (-16.0604, 9.2701) (-16.4011, 9.6824) (-16.7961, 9.9728) (-16.9742, 9.9728) knots 0 0 0 0 1 1 1 1
  spline S78 degree 3 poles (-16.9742, 9.9728) (-17.16, 9.9728) (-17.4136, 9.7076) (-17.4136, 9.4947) knots 0 0 0 0 1 1 1 1
  spline S79 degree 3 poles (-17.4136, 9.4947) (-17.4136, 9.2701) (-17.1426, 9.001) (-16.9045, 8.999) knots 0 0 0 0 1 1 1 1
  line L108 (-16.9045, 8.999) -> (-16.9374, 8.6777)
  spline S80 degree 3 poles (-16.9374, 8.6777) (-17.2955, 8.7106) (-17.6711, 9.1404) (-17.6711, 9.5024) knots 0 0 0 0 1 1 1 1
  spline S81 degree 3 poles (-17.6711, 9.5024) (-17.6711, 9.8683) (-17.2665, 10.2942) (-16.9664, 10.2942) knots 0 0 0 0 1 1 1 1
  spline S82 degree 4 poles (-16.9664, 10.2942) (-16.8135, 10.2942) (-16.5192, 10.1703) (-16.194, 9.8799) (-15.9094, 9.545) knots 0 0 0 0 0 1 1 1 1 1
  spline S83 degree 3 poles (-15.9094, 9.545) (-15.6751, 9.2643) (-15.5067, 9.1055) (-15.4215, 9.0533) knots 0 0 0 0 1 1 1 1
  line L109 (-15.4215, 9.0533) -> (-15.4215, 10.2981)
  spline S84 degree 4 poles (-16.374, 10.633) (-16.8251, 10.633) (-17.3749, 10.8189) (-17.6711, 11.1828) (-17.6711, 11.4616) knots 0 0 0 0 0 1 1 1 1 1
  spline S85 degree 5 poles (-17.6711, 11.4616) (-17.6711, 11.6649) (-17.5066, 11.9746) (-17.1968, 12.174) (-16.7515, 12.2883) (-16.374, 12.2883) knots 0 0 0 0 0 0 1 1 1 1 1 1
  spline S86 degree 4 poles (-16.374, 12.2883) (-15.9268, 12.2883) (-15.377, 12.1044) (-15.0788, 11.7385) (-15.0788, 11.4616) knots 0 0 0 0 0 1 1 1 1 1
  spline S87 degree 2 poles (-15.0788, 11.4616) (-15.0788, 11.0938) (-15.3402, 10.8847) knots 0 0 0 1 1 1
  spline S88 degree 2 poles (-15.3402, 10.8847) (-15.6596, 10.633) (-16.374, 10.633) knots 0 0 0 1 1 1
  spline S89 degree 3 poles (-16.374, 10.9544) (-15.7468, 10.9544) (-15.3344, 11.2467) (-15.3344, 11.4616) knots 0 0 0 0 1 1 1 1
  spline S90 degree 3 poles (-15.3344, 11.4616) (-15.3344, 11.6746) (-15.7487, 11.9669) (-16.374, 11.9669) knots 0 0 0 0 1 1 1 1
  spline S91 degree 3 poles (-16.374, 11.9669) (-17.0013, 11.9669) (-17.4136, 11.6746) (-17.4136, 11.4577) knots 0 0 0 0 1 1 1 1
  spline S92 degree 2 poles (-17.4136, 11.4577) (-17.4136, 11.2428) (-17.2317, 11.1151) knots 0 0 0 1 1 1
  spline S93 degree 2 poles (-17.2317, 11.1151) (-16.9993, 10.9544) (-16.374, 10.9544) knots 0 0 0 1 1 1
  line L110 (-15.1214, 12.749) -> (-17.6614, 12.749)
  line L111 (-17.6614, 12.749) -> (-17.6614, 14.4643)
  line L112 (-17.6614, 14.4643) -> (-17.3614, 14.4643)
  line L113 (-17.3614, 14.4643) -> (-17.3614, 13.0859)
  line L114 (-17.3614, 13.0859) -> (-16.5754, 13.0859)
  line L115 (-16.5754, 13.0859) -> (-16.5754, 14.2785)
  line L116 (-16.5754, 14.2785) -> (-16.2753, 14.2785)
  line L117 (-16.2753, 14.2785) -> (-16.2753, 13.0859)
  line L118 (-16.2753, 13.0859) -> (-15.1214, 13.0859)
  line L119 (-15.1214, 13.0859) -> (-15.1214, 12.749)
  constraints: 1 parallel, 2 other
emboss "Emboss2" sketch "Sketch7" operation add depth 0.0508 direction (0, 0, -1)
equation "\"d19\" = d18"
body "Solid1"
